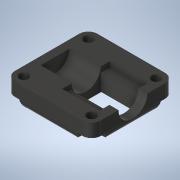
# Autodesk Inventor part: カバー
Saved by Autodesk Inventor 2020 (Build 240168000, 168)
## iProperties
Created: 2020-02-08
Part Number: カバー
Material: 一般
Document SubType Name: Modeling
Designer: 久保寺 真仁
Density: 1 g/cm^3
Appearance: 既定
Author: 久保寺 真仁
Autodesk Inventor part; units mm, degrees
ref_plane "YZ Plane" through (0, 0, 0) normal (1, 0, 0) x (0, 1, 0)
ref_plane "XZ Plane" through (0, 0, 0) normal (0, 1, 0) x (-1, 0, 0)
ref_plane "XY Plane" through (0, 0, 0) normal (0, 0, 1) x (1, 0, 0)
sketch "スケッチ1" plane through (0, 0, 0) normal (0, 0, 1) x (1, 0, 0)
  point P0 (0, 0)
sketch "スケッチ2" plane through (0, 0, 0) normal (0, 1, 0) x (-1, 0, 0)
  line L0 (7.625, 9.25) -> (-7.625, 9.25)
  line L1 (-9.625, 7.25) -> (-9.625, -7.25)
  line L2 (-7.625, -9.25) -> (7.625, -9.25)
  line L3 (9.625, -7.25) -> (9.625, 7.25)
  line L4 (9.625, 9.25) -> (-9.625, -9.25) construction
  line L5 (-9.625, 9.25) -> (9.625, -9.25) construction
  circle A0 centre (7.625, -7.25) radius 1.05
  arc A1 (7.625, -9.25) -> (9.625, -7.25) centre (7.625, -7.25) ccw
  circle A2 centre (7.625, 7.25) radius 1.05
  arc A3 (9.625, 7.25) -> (7.625, 9.25) centre (7.625, 7.25) ccw
  circle A4 centre (-7.625, 7.25) radius 1.05
  circle A5 centre (-7.625, -7.25) radius 1.05
  arc A6 (-7.625, 9.25) -> (-9.625, 7.25) centre (-7.625, 7.25) ccw
  arc A7 (-9.625, -7.25) -> (-7.625, -9.25) centre (-7.625, -7.25) ccw
  point P0 (0, 0)
  dimension "d0" = 19.25
  dimension "d1" = 18.5
  dimension "ねじ穴" = 2.1
  dimension "d6" = 2
  dimension "d7" = 2
  dimension "d8" = 2
  dimension "d9" = 2
  dimension "d10" = 2.1
  dimension "d11" = 2.1
  dimension "d12" = 2.1
  dimension "d13" = 2
  dimension "d14" = 2
  dimension "d15" = 2
  dimension "d16" = 2
  constraints: 12 end point, 8 centre point, 8 point on circle, 4 coincident, 2 midpoint, 2 parallel, 1 horizontal, 1 perpendicular
  measures "d0" distance between parallel lines of L1 L3
  measures "d1" distance between parallel lines of L2 L0
  measures "ねじ穴" diameter of A0
  measures "d6" distance from line of L2 A0.centre
  measures "d7" distance from line of L3 A0.centre
  measures "d8" distance from line of A2.centre L0
  measures "d9" distance from line of A2.centre L3
  measures "d10" diameter of A2
  measures "d11" diameter of A5
  measures "d12" diameter of A4
  measures "d13" distance from line of L1 A4.centre
  measures "d14" distance from line of L0 A4.centre
  measures "d15" distance from line of L1 A5.centre
  measures "d16" distance from line of A5.centre L2
extrude "押し出し1" add sketch "スケッチ2" along normal blind 5
sketch "スケッチ3" plane through (9.625, 0, 7.25) normal (1, 0, 0) x (0, 0, -1)
  line L0 (0, 5) -> (14.5, 5) projected
  circle A0 centre (7.25, 5) radius 3.25
  point P0 (7.25, 0)
  dimension "d19" = 6.5
  constraints: 1 centre point, 1 midpoint
  measures "d19" diameter of A0
extrude "押し出し2" cut sketch "スケッチ3" against normal blind 17.5
sketch "スケッチ4" plane through (0, 0, 0) normal (0, -1, 0) x (1, 0, 0)
  circle A0 centre (-7.625, 7.25) radius 1.05 projected
  circle A1 centre (-7.625, 7.25) radius 2.25
  circle A2 centre (7.625, 7.25) radius 1.05 projected
  circle A3 centre (7.625, 7.25) radius 2.25
  circle A4 centre (7.625, -7.25) radius 1.05 projected
  circle A5 centre (7.625, -7.25) radius 2.25
  circle A6 centre (-7.625, -7.25) radius 1.05 projected
  circle A7 centre (-7.625, -7.25) radius 2.25
  point P0 (0, 0)
  dimension "d22" = 4.5
  dimension "d23" = 4.5
  dimension "d24" = 4.5
  dimension "d25" = 4.5
  constraints: 4 centre point, 4 coincident
  measures "d22" diameter of A1
  measures "d23" diameter of A3
  measures "d24" diameter of A7
  measures "d25" diameter of A5
extrude "押し出し3" cut sketch "スケッチ4" against normal blind 2
fillet "フィレット1" radius 2 4 edges at (0, 0, 9.25) (-9.625, 0, 0) (0, 0, -9.25) (9.625, 0, 0)
sketch "スケッチ5" plane through (0, 0, 0) normal (0, -1, 0) x (1, 0, 0)
  line L0 (-0.875, 3.4) -> (7.625, 3.4)
  line L1 (7.625, 3.4) -> (7.625, -3.4)
  line L2 (7.625, -3.4) -> (-0.875, -3.4)
  line L3 (-0.875, -3.4) -> (-0.875, 3.4)
  line L4 (9.625, 1.25) -> (9.625, 6.2192) projected
  point P0 (0, 0)
  point P1 (-0.875, 0)
  dimension "d29" = 2
  dimension "d30" = 6.8
  dimension "d31" = 8.5
  dimension "d32" = 0
  constraints: 8 end point, 2 parallel, 1 horizontal, 1 midpoint, 1 perpendicular
  measures "d29" distance between parallel lines of L1 L4
  measures "d30" distance between parallel lines of L2 L0
  measures "d31" distance between parallel lines of L1 L3
  measures "d32" vertical distance of point (0, 0) point (-0.875, 0)
extrude "押し出し4" cut sketch "スケッチ5" against normal through all
sketch "スケッチ6" plane through (0, 5, 0) normal (0, 1, 0) x (1, 0, 0)
  line L0 (7.625, -5.4) -> (-0.875, -5.4)
  line L1 (-0.875, -5.4) -> (-0.875, 5.4)
  line L2 (-0.875, 5.4) -> (7.625, 5.4)
  line L3 (7.625, 5.4) -> (7.625, -5.4)
  line L4 (9.625, -7.25) -> (9.625, -3.25) projected
  point P0 (0, 0)
  point P1 (-0.875, 0)
  point P2 (-0.875, -3.4)
  point P3 (7.625, -3.4)
  dimension "d35" = 2
  dimension "d36" = 8.5
  dimension "d37" = 10.8
  dimension "d38" = 0
  dimension "d39" = 8.5
  constraints: 8 end point, 2 parallel, 1 horizontal, 1 midpoint, 1 perpendicular
  measures "d35" distance between parallel lines of L3 L4
  measures "d36" distance of L0.start L0.end
  measures "d37" distance between parallel lines of L2 L0
  measures "d38" vertical distance of point (-0.875, 0) point (0, 0)
  measures "d39" distance of point (-0.875, -3.4) point (7.625, -3.4)
extrude "押し出し5" cut sketch "スケッチ6" against normal blind 1.25
equation "\"d7\" = d6"
equation "\"d8\" = d6"
equation "\"d9\" = d6"
equation "\"d10\" = ねじ穴"
equation "\"d11\" = ねじ穴"
equation "\"d12\" = ねじ穴"
equation "\"d13\" = d6"
equation "\"d14\" = d6"
equation "\"d15\" = d6"
equation "\"d16\" = d6"
equation "\"d23\" = d22"
equation "\"d24\" = d22"
equation "\"d25\" = d22"
equation "\"d36\" = d39"
